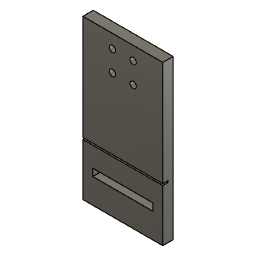
Tube Test Assembly v8 (Autodesk Fusion 360 archive; units mm, degrees)
design "Tube Back Plate"
Autodesk Fusion 360 part; units mm, degrees
sketch "Sketch1" plane through (0, 0, 0) normal (0, 0, 1) x (1, 0, 0)
  line L0 (0, 0) -> (77, 0)
  line L1 (77, 0) -> (77, 153)
  line L2 (77, 153) -> (0, 153)
  line L3 (0, 153) -> (0, 0)
  circle A0 centre (28.5, 140) radius 3.05
  circle A1 centre (48.5, 140) radius 3.05
  circle A2 centre (28.5, 120) radius 3.05
  circle A3 centre (48.5, 120) radius 3.05
  line L4 (9.5, 31) -> (67.5, 31)
  line L5 (67.5, 31) -> (67.5, 24)
  line L6 (67.5, 24) -> (9.5, 24)
  line L7 (9.5, 24) -> (9.5, 31)
  dimension "d1" = 153
  dimension "d2" = 77
  dimension "d3" = 6.1
  dimension "d4" = 6.1
  dimension "d5" = 6.1
  dimension "d6" = 6.1
  dimension "d7" = 140
  dimension "d8" = 140
  dimension "d9" = 120
  dimension "d10" = 120
  dimension "d11" = 20
  dimension "d12" = 20
  dimension "d13" = 28.5
  dimension "d14" = 28.5
  dimension "d17" = 24
  dimension "d18" = 9.5
  dimension "d19" = 9.5
  dimension "d20" = 7
  constraint horizontal L0
  constraint vertical L1
  constraint horizontal L2
  constraint vertical L3
  constraint coincident L0.start L3.end
  constraint horizontal L4
  constraint vertical L5
  constraint horizontal L6
  constraint vertical L7
  measures "d1" distance of L0.start L2.end
  measures "d2" distance of L1.end L2.end
  measures "d3" diameter of A0
  measures "d4" diameter of A1
  measures "d5" diameter of A2
  measures "d6" diameter of A3
  measures "d7" distance of L0 A0.centre
  measures "d8" distance of L0 A1.centre
  measures "d9" distance of L0 A3.centre
  measures "d10" distance of L0 A2.centre
  measures "d11" distance of A0.centre A1.centre
  measures "d12" distance of A2.centre A3.centre
  measures "d13" distance of L1 A1.centre
  measures "d14" distance of L1 A3.centre
  measures "d17" distance of L0 L6
  measures "d18" distance of L3 L6.end
  measures "d19" distance of L1 L5
  measures "d20" distance of L4.start L6.end
extrude "Extrude1" add sketch "Sketch1" along normal blind 10
sketch "Sketch2" plane through (0, 0, 10) normal (0, 0, 1) x (1, 0, 0)
  circle A0 centre (28.5, 120) radius 3.05
  circle A1 centre (48.5, 120) radius 3.05
  circle A2 centre (48.5, 140) radius 3.05
  circle A3 centre (28.5, 140) radius 3.05
  line L0 (67.5, 24) -> (9.5, 24)
  line L1 (9.5, 24) -> (9.5, 31)
  line L2 (9.5, 31) -> (67.5, 31)
  line L3 (67.5, 31) -> (67.5, 24)
  line L4 (0, 153) -> (0, 0)
  line L5 (0, 0) -> (77, 0)
  line L6 (77, 0) -> (77, 153)
  line L7 (77, 153) -> (0, 153)
  line L8 (0, 51.8) -> (77, 51.8)
  line L9 (77, 51.8) -> (77, 50.2)
  line L10 (77, 50.2) -> (0, 50.2)
  line L11 (0, 50.2) -> (0, 51.8)
  dimension "d21" = 50.2
  dimension "d22" = 51.8
  constraint horizontal L8
  constraint vertical L9
  constraint horizontal L10
  constraint vertical L11
  constraint coincident L6 L9.end
  constraint coincident L4 L8.start
  measures "d21" distance of L5 L10
  measures "d22" distance of L5 L8
extrude "Extrude2" cut sketch "Sketch2" against normal blind 5 contours L4 L6 L8 L9 L10 L11
equation "d4 = d3"
equation "d5 = d3"
equation "d6 = d3"
equation "d8 = d7"
equation "d10 = d9"
equation "d12 = d11"
equation "d14 = d13"

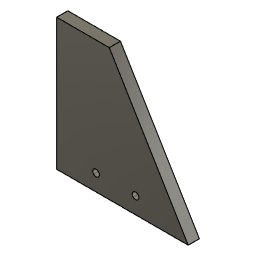
design "Tube Supporter"
Autodesk Fusion 360 part; units mm, degrees
sketch "Sketch1" plane through (0, 0, 0) normal (0, 0, 1) x (1, 0, 0)
  line L0 (0, 0) -> (0, 100)
  line L1 (0, 100) -> (40, 100)
  line L2 (40, 100) -> (100, 0)
  line L3 (100, 0) -> (0, 0)
  circle A0 centre (30, 12.5) radius 2.55
  circle A1 centre (60, 12.5) radius 2.55
  dimension "d3" = 40
  dimension "d4" = 100
  dimension "d5" = 100
  dimension "d14" = 12.5
  dimension "d15" = 12.5
  dimension "d16" = 5.1
  dimension "d17" = 5.1
  dimension "d18" = 30
  dimension "d19" = 30
  constraint coincident L0.start L3.end
  constraint vertical L0
  constraint perpendicular L0 L1
  constraint perpendicular L0 L3
  measures "d3" distance of L0.end L1.end
  measures "d4" distance of L0.start L0.end
  measures "d5" distance of L0.start L2.end
  measures "d14" distance of L3 A0.centre
  measures "d15" distance of L3 A1.centre
  measures "d16" diameter of A0
  measures "d17" diameter of A1
  measures "d18" distance of A0.centre A1.centre
  measures "d19" distance of L0 A0.centre
extrude "Extrude1" add sketch "Sketch1" along normal blind 8.5
equation "d15 = d14"
equation "d17 = d16"

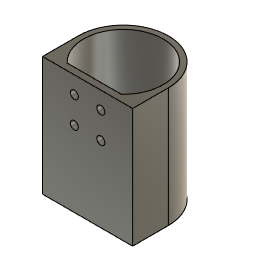
design "Tube"
Autodesk Fusion 360 part; units mm, degrees
sketch "Sketch1" plane through (0, 0, 0) normal (0, 0, 1) x (1, 0, 0)
  circle A0 centre (0, 0) radius 30
  circle A1 centre (0, 0) radius 34
  line L0 (0, 30) -> (0, -22) construction
  line L1 (-20.3961, -22) -> (20.3961, -22)
  line L2 (-34, -27) -> (34, -27)
  line L3 (-34, -27) -> (-34, 0)
  line L4 (34, -27) -> (34, 0)
  circle A2 centre (0, 4) radius 25.4 construction
  dimension "d1" = 60
  dimension "d2" = 68
  dimension "d3" = 52
  dimension "d6" = 5
  dimension "d38" = 50.8
  constraint coincident A0.centre A1.centre
  constraint coincident A0 L0.start
  constraint vertical L0
  constraint coincident A0.centre L0
  constraint coincident A0 L1.start
  constraint coincident A0 L1.end
  constraint horizontal L1
  constraint coincident L0.end L1
  constraint parallel L1 L2
  constraint coincident A1 L3.end
  constraint tangent A1 L3
  constraint coincident A1 L4.end
  constraint tangent A1 L4
  constraint vertical L4
  constraint vertical L3
  constraint midpoint L0 A2.centre
  measures "d1" diameter of A0
  measures "d2" diameter of A1
  measures "d3" distance of L0.start L0.end
  measures "d6" vertical distance of L1.start L2.start
  measures "d38" diameter of A2
extrude "Extrude1" add sketch "Sketch1" along normal blind 90 contours A0 A1 L2 | A0 L1 L2 | A1 L2 L3 | A1 L2 L4 picked at (-32.5234, 2.2674)
sketch "Sketch8" plane through (0, -27, 0) normal (0, -1, 0) x (1, 0, 0)
  line L0 (-34, 0) -> (34, 0)
  line L1 (34, 0) -> (34, 90)
  line L2 (34, 90) -> (-34, 90)
  line L3 (-34, 90) -> (-34, 0)
  circle A0 centre (-10, 77) radius 3.05
  circle A1 centre (10, 77) radius 3.05
  circle A2 centre (-10, 57) radius 3.05
  circle A3 centre (10, 57) radius 3.05
  dimension "d43" = 6.1
  dimension "d44" = 6.1
  dimension "d45" = 6.1
  dimension "d46" = 6.1
  dimension "d47" = 13
  dimension "d48" = 13
  dimension "d49" = 33
  dimension "d50" = 33
  dimension "d51" = 20
  dimension "d52" = 20
  dimension "d53" = 24
  dimension "d54" = 24
  measures "d43" diameter of A0
  measures "d44" diameter of A1
  measures "d45" diameter of A2
  measures "d46" diameter of A3
  measures "d47" distance of L2 A0.centre
  measures "d48" distance of L2 A1.centre
  measures "d49" distance of L2 A2.centre
  measures "d50" distance of L2 A3.centre
  measures "d51" distance of A0.centre A1.centre
  measures "d52" distance of A2.centre A3.centre
  measures "d53" distance of L1 A1.centre
  measures "d54" distance of L1 A3.centre
extrude "Extrude10" cut sketch "Sketch8" against normal blind 5 contours A0 | A1 | A2 | A3
equation "d44 = d43"
equation "d45 = d43"
equation "d46 = d43"
equation "d48 = d47"
equation "d50 = d49"
equation "d52 = d51"
equation "d54 = d53"
